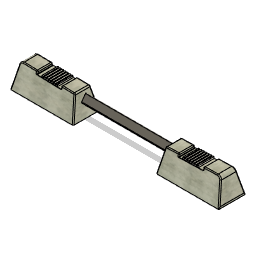
B440 NP Sleeper (Autodesk Fusion 360 design; units mm, degrees)
Autodesk Fusion 360 part; units mm, degrees
sketch "Sketch1" plane through (0, 0, 0) normal (0, 1, 0) x (1, 0, 0)
  line L0 (0, 0) -> (0, 145) construction
  line L1 (0, 145) -> (220, 145) construction
  line L2 (220, 145) -> (220, -145) construction
  line L3 (220, -145) -> (0, -145) construction
  line L4 (0, -145) -> (0, 0) construction
  line L5 (220, 0) -> (220, 90)
  line L6 (220, 0) -> (220, -90)
  line L7 (0, 145) -> (0, -145)
  line L8 (220, -90) -> (0, -145)
  line L9 (0, 145) -> (220, 90)
  line L10 (0, -145) -> (291.0428, -72.2393)
  line L11 (0, 145) -> (291.0428, 72.2393)
  line L12 (291.0428, -72.2393) -> (291.0428, -77.6398)
  line L13 (291.0428, -77.6398) -> (291.0428, -145)
  line L14 (0, -145) -> (291.0428, -145)
  line L15 (0, 145) -> (291.0428, 145)
  line L16 (291.0428, 72.2393) -> (291.0428, 145)
  dimension "d7" = 145
  dimension "d8" = 220
  dimension "d10" = 220
  dimension "d11" = 90
  dimension "d12" = 90
  dimension "d33" = 300
  constraint coincident L0.start L4.end
  constraint perpendicular L3 L4
  constraint midpoint L2 L5.start
  constraint perpendicular L3 L7
  constraint parallel L8 L10
  constraint parallel L12 L13
  constraint perpendicular L4 L14
  constraint perpendicular L0 L15
  constraint vertical L16
  measures "d7" distance of L0.start L0.end
  measures "d8" distance of L0.end L1.end
  measures "d10" distance of L2.end L3.end
  measures "d11" distance of L5.start L5.end
  measures "d12" distance of L5.start L6.end
  measures "d33" distance of L0.end L11.end
sketch "Sketch2" plane through (0, 0, 0) normal (0, 0, 1) x (1, 0, 0)
  line L0 (0, 0) -> (0, 680)
  line L1 (0, 680) -> (20, 680)
  line L2 (261, 770) -> (261, -100) construction
  line L3 (220, 770) -> (220, -100) construction
  line L4 (410, 320) -> (-140, 320) construction
  line L5 (20, 680) -> (261, 637.5052)
  line L6 (20, 680) -> (320, 680) construction
  line L7 (0, 0) -> (246, 43.3764)
  line L8 (0, 0) -> (353.5534, 0) construction
  line L9 (239.2572, 320) -> (347.9817, 320) construction
  line L10 (261.8314, 448.025) -> (261, 448.1716)
  line L11 (246, 770) -> (246, -100) construction
  line L12 (252.9839, 320) -> (401.4575, 320) construction
  line L13 (252.9839, 320) -> (121.2329, 323.3263) construction
  line L14 (256.265, 449.9586) -> (124.514, 453.2849) construction
  line L15 (251.3431, 190) -> (117.9518, 193.3677) construction
  line L16 (251.3431, 190) -> (401.4575, 190) construction
  line L17 (220, 190.7913) -> (226.5621, 450.7085)
  line L18 (256.265, 449.9586) -> (226.5621, 450.7085)
  line L19 (251.3431, 190) -> (220, 190.7913)
  line L20 (246, 43.3764) -> (249.7029, 190.0414)
  line L21 (256.265, 449.9586) -> (261, 637.5052)
  dimension "d15" = 680
  dimension "d16" = 20
  dimension "d17" = 261
  dimension "d18" = 220
  dimension "d19" = 360
  dimension "d21" = 10
  dimension "d22" = 10
  dimension "d26" = 15
  dimension "d28" = 130
  dimension "d29" = 130
  constraint coincident L0.start L7.start
  constraint vertical L2
  constraint vertical L3
  constraint horizontal L4
  constraint horizontal L6
  constraint coincident L2 L5.end
  constraint horizontal L8
  constraint coincident L4 L9.start
  constraint horizontal L9
  constraint coincident L2 L10.end
  constraint vertical L11
  constraint coincident L11 L7.end
  constraint coincident L9 L12.start
  constraint horizontal L12
  constraint perpendicular L13 L20
  constraint coincident L15 L17.start
  constraint coincident L3 L17.start
  constraint perpendicular L15 L17
  constraint coincident L14 L17.end
  constraint perpendicular L17 L18
  constraint parallel L15 L19
  constraint collinear L20 L21
  constraint coincident L15 L20.end
  measures "d15" distance of L0.start L0.end
  measures "d16" distance of L0.end L1.end
  measures "d17" distance of L0 L2
  measures "d18" distance of L0 L3
  measures "d19" distance of L1 L4
  measures "d21" angle of L5 L6
  measures "d22" angle of L7 L8
  measures "d26" distance of L2 L11
extrude "Extrude3" add sketch "Sketch2" along normal mid plane 290 makes body 1
extrude "Extrude4" cut sketch "Sketch1" along normal through all contours L9 L11 L15 L16 | L8 L10 L12 L13 L14 bodies 1
fillet "Fillet1" radius 40 1 edges at (261, 637.5052, 0) on bodies 1
fillet "Fillet2" radius 15 1 edges at (246, 43.3764, 0) on bodies 1
fillet "Fillet3" radius 10 12 edges at (116.9596, 20.6231, -115.7601) (242.6825, 46.2323, -84.3294) (248.0062, 122.8406, -82.9984) (248.0062, 122.8406, 82.9984) (242.6825, 46.2323, 84.3294) (116.9596, 20.6231, 115.7601) (258.198, 526.5206, -80.4505) (251.1075, 629.4149, -82.2231) (123.5448, 661.7423, -114.1138) (123.5448, 661.7423, 114.1138) (251.1075, 629.4149, 82.2231) (258.198, 526.5206, 80.4505) on bodies 1
fillet "Fillet4" radius 10 10 edges at (231.0649, 190.512, -87.2338) (247.5853, 190.0949, -80.9203) (249.7029, 190.0414, 0) (247.5853, 190.0949, 80.9203) (231.0649, 190.512, 87.2338) (237.6271, 450.4291, -85.5932) (254.1475, 450.012, -79.2797) (256.265, 449.9586, 0) (254.1475, 450.012, 79.2797) (237.6271, 450.4291, 85.5932) on bodies 1
fillet "Fillet5" radius 3 6 edges at (219.9266, 187.8849, -87.0215) (220, 190.7913, 0) (219.9266, 187.8849, 87.0215) (226.6366, 453.6582, -85.2994) (226.5621, 450.7085, 0) (226.6366, 453.6582, 85.2994) on bodies 1
fillet "Fillet6" radius 2 6 edges at (227.5472, 457.558, 88.1132) (223.2827, 320.8156, 89.1793) (220.5611, 184.2751, 89.8597) (220.6251, 184.0769, -89.8437) (223.2827, 320.8156, -89.1793) (227.4544, 457.3154, -88.1364) on bodies 1
sketch "Sketch3" plane through (0, 0, 0) normal (0, 1, 0) x (1, 0, 0)
  line L0 (20, 130.1264) -> (20, -130.1264)
  line L1 (0, 0) -> (380, 0) construction
  line L2 (0, 0) -> (0, 333.0776) construction
  line L3 (85, 0) -> (85, 333.0776) construction
  line L4 (85, -60) -> (205, -60) construction
  line L5 (205, -60) -> (205, 60) construction
  line L6 (205, 60) -> (85, 60) construction
  line L7 (85, 60) -> (85, -60) construction
  line L8 (205, 60) -> (85, -60) construction
  line L9 (205, -60) -> (85, 60) construction
  line L10 (225.6218, 59.4086) -> (123.0914, -43.1218) construction
  line L11 (169.0063, -45.2195) -> (82.6711, 41.1157) construction
  line L12 (145, -21.2132) -> (205, 38.7868) construction
  line L13 (145, -21.2132) -> (85, 38.7868) construction
  line L14 (95, 50) -> (95, -50) construction
  line L15 (95, -50) -> (195, -50) construction
  line L16 (195, -50) -> (195, 50) construction
  line L17 (195, 50) -> (95, 50) construction
  line L18 (189.7168, 34.1102) -> (139.6967, -15.9099)
  arc A0 (139.6967, -15.9099) -> (150.3033, -26.5165) centre (145, -21.2132) ccw
  line L19 (150.3033, -26.5165) -> (200.3234, 23.5036)
  arc A1 (200.3234, 23.5036) -> (189.7168, 34.1102) centre (195.0201, 28.8069) ccw
  line L20 (195.0201, 28.8069) -> (145, -21.2132) construction
  line L21 (150.3033, -15.9099) -> (100.3033, 34.0901)
  arc A2 (100.3033, 34.0901) -> (89.6967, 23.4835) centre (95, 28.7868) ccw
  line L22 (89.6967, 23.4835) -> (139.6967, -26.5165)
  arc A3 (139.6967, -26.5165) -> (150.3033, -15.9099) centre (145, -21.2132) ccw
  line L23 (145, -21.2132) -> (95, 28.7868) construction
  dimension "d41" = 85
  dimension "d44" = 120
  dimension "d45" = 120
  dimension "d46" = 15
  dimension "d47" = 15
  dimension "d48" = 10
  dimension "d49" = 15
  dimension "d50" = 15
  constraint coincident L1.start L2.start
  constraint perpendicular L0 L1
  constraint perpendicular L1 L2
  constraint horizontal L4
  constraint vertical L5
  constraint horizontal L6
  constraint vertical L7
  constraint parallel L8 L10
  constraint parallel L9 L11
  constraint coincident L10 L12.end
  constraint coincident L5 L12.end
  constraint perpendicular L11 L12
  constraint coincident L11 L12.start
  constraint coincident L11 L13.end
  constraint coincident L7 L13.end
  constraint coincident L3 L13.end
  constraint coincident L12.start L13.start
  constraint tangent L18 A0
  constraint tangent A0 L19
  constraint parallel L18 L19
  constraint tangent L19 A1
  constraint tangent L18 A1
  constraint perpendicular L11 L20
  constraint tangent L21 A2
  constraint tangent A2 L22
  constraint parallel L21 L22
  constraint tangent L22 A3
  constraint tangent L21 A3
  constraint coincident L11 A2.centre
  constraint coincident L14 A2.centre
  measures "d44" distance of L4.start L4.end
  measures "d45" distance of L4.start L6.end
  measures "d46" distance of L8 L10
  measures "d47" distance of L9 L11
  measures "d49" diameter of A0
  measures "d50" diameter of A2
ref_plane "WorkPlane3" through (0, -450, 0) normal (0, 1, 0) x (0, 0, 1)
mirror "Mirror1" about plane through (0, -450, 0) normal (0, 1, 0) of bodies 1 makes body 2
extrude "Extrude6" add sketch "Sketch3" along normal up to surface and the other way up to surface separate body end surface through (0, 0, 0) normal (0.173648, -0.984808, 0) offset 0 second end surface through (0, -900, 0) normal (0.173648, 0.984808, 0) offset 0 makes body 3
ref_plane "WorkPlane4" through (234.6336, 320.4633, 0) normal (0.025239, 0.999681, 0) x (-0.999681, 0.025239, 0)
ref_plane "WorkPlane5" through (234.6336, -1220.4633, 0) normal (0.025239, -0.999681, 0) x (-0.999681, -0.025239, 0)
sketch "Sketch4" plane through (215.046, -5.4293, 0) normal (0.999681, -0.025239, 0) x (0, 0, -1)
  line L0 (88.4432, 195.5118) -> (86.7922, 457.1672)
  ellipse E0 centre (77.2388, 466.2831) end of major axis (90.6387, 466.2831) minor radius 13 (77.2388, 453.2831) -> (86.7922, 457.1672) ccw
  line L1 (77.2388, 453.2831) -> (-77.2388, 453.2831)
  ellipse E1 centre (-77.2388, 466.2831) end of major axis (-90.6387, 466.2831) minor radius 13 (-86.7922, 457.1672) -> (-77.2388, 453.2831) ccw
  line L2 (-86.7922, 457.1672) -> (-88.4432, 195.5118)
  ellipse E2 centre (-79.0056, 186.2831) end of major axis (-92.4054, 186.2831) minor radius 13 (-79.0056, 199.2831) -> (-88.4432, 195.5118) ccw
  line L3 (-79.0056, 199.2831) -> (79.0056, 199.2831)
  ellipse E3 centre (79.0056, 186.2831) end of major axis (92.4054, 186.2831) minor radius 13 (88.4432, 195.5118) -> (79.0056, 199.2831) ccw
  line L4 (0, 453.2831) -> (0, 199.2831) construction
  line L5 (-87.6177, 326.3395) -> (87.6177, 326.3395) construction
  line L6 (-87.6177, 236.3395) -> (87.6177, 236.3395) construction
  line L7 (-87.6177, 404.8395) -> (87.6177, 404.8395) construction
  line L8 (-85.7933, 404.8395) -> (85, 404.8395)
  line L9 (85, 404.8395) -> (85, 236.3395)
  line L10 (85, 236.3395) -> (-85.7933, 236.3395)
  line L11 (-85.7933, 236.3395) -> (-85.7933, 404.8395)
  dimension "d67" = 90
  dimension "d68" = 78.5
  constraint midpoint L1 L4.start
  constraint midpoint L3 L4.end
  constraint midpoint L2 L5.start
  constraint midpoint L0 L5.end
  constraint perpendicular L8 L9
  constraint parallel L8 L10
  constraint parallel L9 L11
  constraint coincident L7 L8.end
  constraint parallel L7 L8
extrude "Extrude7" add sketch "Sketch4" along normal blind 18 separate body contours L8 L9 L10 L11 makes body 4
sketch "Sketch5" plane through (0, 0, 85.7933) normal (0, 0, 1) x (1, 0, 0)
  line L0 (225.2638, 399.2813) -> (221.011, 230.835)
  line L1 (221.011, 230.835) -> (239.0052, 230.3807)
  line L2 (239.0052, 230.3807) -> (243.258, 398.827)
  line L3 (243.258, 398.827) -> (225.2638, 399.2813)
  line L4 (234.2609, 399.0541) -> (230.0081, 230.6078) construction
  line L5 (233.9156, 385.3785) -> (244.2794, 385.1169)
  line L6 (244.2794, 385.1169) -> (244.027, 375.1201)
  line L7 (244.027, 375.1201) -> (233.6632, 375.3817)
  line L8 (233.9156, 385.3785) -> (233.6632, 375.3817)
  line L9 (233.2493, 358.987) -> (232.9969, 348.9901)
  line L10 (243.613, 358.7253) -> (243.3607, 348.7285)
  line L11 (233.2493, 358.987) -> (243.613, 358.7253)
  line L12 (243.3607, 348.7285) -> (232.9969, 348.9901)
  line L13 (232.583, 332.5954) -> (232.3306, 322.5985)
  line L14 (242.9467, 332.3337) -> (242.6943, 322.3369)
  line L15 (232.583, 332.5954) -> (242.9467, 332.3337)
  line L16 (242.6943, 322.3369) -> (232.3306, 322.5985)
  line L17 (231.9167, 306.2038) -> (231.6643, 296.207)
  line L18 (242.2804, 305.9421) -> (242.028, 295.9453)
  line L19 (231.9167, 306.2038) -> (242.2804, 305.9421)
  line L20 (242.028, 295.9453) -> (231.6643, 296.207)
  line L21 (231.2504, 279.8122) -> (230.998, 269.8154)
  line L22 (241.6141, 279.5505) -> (241.3617, 269.5537)
  line L23 (231.2504, 279.8122) -> (241.6141, 279.5505)
  line L24 (241.3617, 269.5537) -> (230.998, 269.8154)
  line L25 (230.5841, 253.4206) -> (230.3317, 243.4238)
  line L26 (240.9478, 253.1589) -> (240.6954, 243.1621)
  line L27 (230.5841, 253.4206) -> (240.9478, 253.1589)
  line L28 (240.6954, 243.1621) -> (230.3317, 243.4238)
  dimension "d71" = 10
  dimension "d74" = 132
  dimension "d75" = 0
  constraint midpoint L3 L4.start
  constraint midpoint L1 L4.end
  constraint coincident L4 L5.start
  constraint perpendicular L2 L5
  constraint coincident L4 L7.end
  constraint perpendicular L4 L7
  measures "d71" distance of L5.end L6.end
extrude "Extrude8" cut sketch "Sketch5" against normal through all contours L2 L5 L7 L8 | L2 L25 L27 L28 | L2 L9 L11 L12 | L2 L21 L23 L24 | L2 L13 L15 L16 | L2 L17 L19 L20 bodies 4
mirror "Mirror2" about plane through (0, -450, 0) normal (0, 1, 0) of bodies 4 makes body 5
move_body "Move1" bodies 1 4 5 2 3 to x (0, 1, 0) y (-1, 0, 0) z (0, 0, 1) at (419.7506, -59.1567, 0)
ref_plane "WorkPlane6" through (869.7506, 98.9771, 0) normal (-1, 0, 0) x (0, 1, 0)
move_body "Move2" bodies 2 5 3 1 4 to x (1, 0, 0) y (0, 1, 0) z (0, 0, 1) at (-869.4566, -21.9512, -5.4878)
equation "d7 = ( 290 / 2 ) * 1 mm"
equation "d11 = ( 180 / 2 ) * 1 mm"
equation "d12 = ( 180 / 2 ) * 1 mm"
equation "d30 = ( 290 / 2 ) * 1 mm"
named bodies: "Concrete (1)", "Concrete (2)", "C-Steel", "Selle (1)", "Selle (1) (1)"
